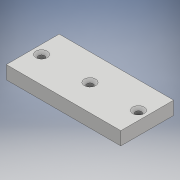
# Autodesk Inventor part: Part03
Saved by Autodesk Inventor 2018 (Build 220112000, 112)
## iProperties
Created: 2019-02-06
Part Number: Part03
Material: Generic
Document SubType Name: Modeling
Designer: JARVIS
Density: 1 g/cm^3
Appearance: Default
Author: JARVIS
Autodesk Inventor part; units mm, degrees
ref_plane "YZ Plane" through (0, 0, 0) normal (1, 0, 0) x (0, 1, 0)
ref_plane "XZ Plane" through (0, 0, 0) normal (0, 1, 0) x (-1, 0, 0)
ref_plane "XY Plane" through (0, 0, 0) normal (0, 0, 1) x (1, 0, 0)
sketch "Sketch1" plane through (0, 0, 0) normal (0, 0, 1) x (1, 0, 0)
  line L0 (-32.5, 15) -> (32.5, 15)
  line L1 (32.5, 15) -> (32.5, -15)
  line L2 (32.5, -15) -> (-32.5, -15)
  line L3 (-32.5, -15) -> (-32.5, 15)
  circle A0 centre (0, 0) radius 1.75
  circle A1 centre (-27.5, 0) radius 1.75
  circle A2 centre (27.5, 0) radius 1.75
  point P0 (0, 15)
  point P1 (32.5, 0)
  dimension "d0" = 65
  dimension "d1" = 30
  dimension "d2" = 3.5
  dimension "d3" = 5
  dimension "d4" = 5
  constraints: 8 end point, 3 centre point, 3 horizontal alignment, 2 equal radius, 2 midpoint, 2 parallel, 1 coincident, 1 horizontal, 1 perpendicular, 1 vertical alignment
  measures "d0" distance of L0.start L0.end
  measures "d1" distance of L2.end L0.start
  measures "d2" diameter of A2
  measures "d3" distance from line of L3 A1.centre
  measures "d4" distance of point (32.5, 0) A2.centre
extrude "Extrusion1" add sketch "Sketch1" along normal blind 7.5
chamfer "Chamfer1" distance 1.5 angle 45 3 edges at (-29.25, 0, 7.5) (-1.75, 0, 7.5) (25.75, 0, 7.5)
body "Solid1"
